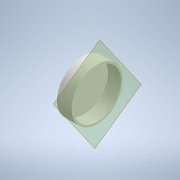
# Autodesk Inventor part: Part11
Saved by Autodesk Inventor 2020 (Build 240168000, 168)
## iProperties
Created: 2022-04-08
Part Number: Part11
Material: Generic
Document SubType Name: Modeling
Designer: Mic
Density: 1 g/cm^3
Appearance: Default
Author: Mic
Autodesk Inventor part; units mm, degrees
ref_plane "YZ Plane" through (0, 0, 0) normal (1, 0, 0) x (0, 1, 0)
ref_plane "XZ Plane" through (0, 0, 0) normal (0, 1, 0) x (-1, 0, 0)
ref_plane "XY Plane" through (0, 0, 0) normal (0, 0, 1) x (1, 0, 0)
ref_plane "Work Plane1" through (-4.4612, 13.9347, 31.1596) normal (-1, 0, 0) x (0, -0.5741, 0.8188)
sketch "Sketch1" plane through (-4.4612, 13.9347, 31.1596) normal (-1, 0, 0) x (0, -0.5741, 0.8188)
  circle A0 centre (0, 0) radius 16.4653 construction
  arc A1 (-8.9965, -1.0986) -> (8.4267, -3.3371) centre (0, 0) ccw construction
  line L0 (-8.9965, -1.0986) -> (-3.439, -1.0986) construction
  arc A2 (-3.439, -1.0986) -> (1.3777, -3.3371) centre (0, 0) ccw construction
  line L1 (1.3777, -3.3371) -> (8.4267, -3.3371) construction
  line L2 (8.4267, 3.3371) -> (1.3777, 3.3371) construction
  arc A3 (1.3777, 3.3371) -> (-3.439, 1.0986) centre (0, 0) ccw construction
  line L3 (-3.439, 1.0986) -> (-8.9965, 1.0986) construction
  arc A4 (8.4267, 3.3371) -> (-8.9965, 1.0986) centre (0, 0) ccw construction
  arc A5 (-7.3545, -6.9867) -> (-10.7722, -10.2334) centre (-9.0634, -8.61) ccw construction
  arc A6 (-7.3545, -6.9867) -> (6.7299, -7.5902) centre (0, 0) ccw construction
  arc A7 (9.8573, -11.1174) -> (6.7299, -7.5902) centre (8.2936, -9.3538) ccw construction
  arc A8 (-10.7722, -10.2334) -> (9.8573, -11.1174) centre (0, 0) ccw construction
  arc A9 (6.7299, 7.5902) -> (-7.3545, 6.9867) centre (0, 0) ccw construction
  arc A10 (-10.7722, 10.2334) -> (-7.3545, 6.9867) centre (-9.0634, 8.61) ccw construction
  arc A11 (9.8573, 11.1174) -> (-10.7722, 10.2334) centre (0, 0) ccw construction
  arc A12 (6.7299, 7.5902) -> (9.8573, 11.1174) centre (8.2936, 9.3538) ccw construction
  line L4 (1.6496, 2.4654) -> (13.6732, 2.4654) construction
  arc A13 (13.6732, -2.4654) -> (13.6732, 2.4654) centre (0, 0) ccw construction
  line L5 (13.6732, -2.4654) -> (1.6496, -2.4654) construction
  arc A14 (1.6496, 2.4654) -> (1.6496, -2.4654) centre (0, 0) ccw construction
  circle A15 centre (0, 0) radius 16.4653
  circle A16 centre (0, 0) radius 15.2389
  point P0 (-17.5128, -29.2984)
  constraints: 2 centre point, 2 coincident, 1 concentric
extrude "Extrusion1" add sketch "Sketch1" along normal blind 9.327
sketch "Sketch2" plane through (-13.7882, 13.9347, 31.1596) normal (-1, 0, 0) x (0, 0, 1)
  circle A0 centre (0, 0) radius 16.4653 projected
  circle A1 centre (0, 0) radius 15.2389 projected
  point P0 (-31.1596, -13.9347)
extrude "Extrusion2" add sketch "Sketch2" against normal blind 1 contours A1
body "Solid1"
